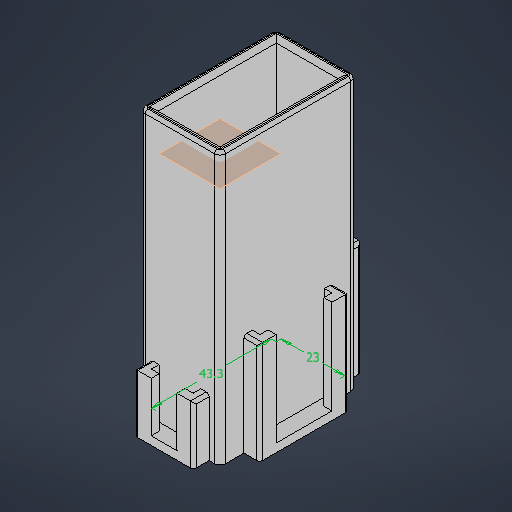
# Autodesk Inventor part: cajaPilas
Saved by Autodesk Inventor 2026.2 (Build 302298010, 298A)
## iProperties
Created: 2026-08-19
Part Number: cajaPilas
Material: Genérico
Document SubType Name: Modeling
Designer: samue
Density: 1 g/cm^3
Appearance: Valor por defecto
Author: samue
Autodesk Inventor part; units mm, degrees
ref_plane "YZ Plane" through (0, 0, 0) normal (1, 0, 0) x (0, 1, 0)
ref_plane "XZ Plane" through (0, 0, 0) normal (0, 1, 0) x (-1, 0, 0)
ref_plane "XY Plane" through (0, 0, 0) normal (0, 0, 1) x (1, 0, 0)
sketch "Boceto1" plane through (0, 0, 0) normal (0, 1, 0) x (-1, 0, 0)
  line L0 (0, 0) -> (23, 0)
  line L1 (23, 0) -> (23, -43.3)
  line L2 (23, -43.3) -> (0, -43.3)
  line L3 (0, -43.3) -> (0, 0)
  dimension "d0" = 23
  dimension "d1" = 43.3
  constraints: 8 end point, 2 parallel, 1 horizontal, 1 perpendicular
  measures "d0" distance of L1.end L2.end
  measures "d1" distance of L0.end L1.end
ref_plane "Plano de trabajo1" through (0, 92, 0) normal (0, 1, 0) x (1, 0, 0)
sketch "Boceto2" plane through (0, 92, 0) normal (0, 1, 0) x (1, 0, 0)
  line L0 (0, 43.3) -> (-23, 43.3) projected
  line L1 (-23, 43.3) -> (-23, 0) projected
  line L2 (-23, 0) -> (0, 0) projected
  line L3 (0, 0) -> (0, 43.3) projected
  line L4 (-26, -1) -> (-26, 44.3)
  line L5 (-24, 46.3) -> (1, 46.3)
  line L6 (3, 44.3) -> (3, -1)
  line L7 (1, -3) -> (-24, -3)
  arc A0 (-26, -1) -> (-24, -3) centre (-24, -1) ccw
  arc A1 (1, -3) -> (3, -1) centre (1, -1) ccw
  arc A2 (3, 44.3) -> (1, 46.3) centre (1, 44.3) ccw
  arc A3 (-24, 46.3) -> (-26, 44.3) centre (-24, 44.3) ccw
  point P0 (-11.5, 21.65)
  point P1 (-26, -3)
  point P2 (-26, 46.3)
  point P3 (3, 46.3)
  point P4 (3, -3)
  dimension "d4" = 21.65
  dimension "d5" = 11.5
  dimension "d6" = 3
  dimension "d9" = 2
  constraints: 8 end point, 8 point on circle, 8 point on line, 8 tangent, 4 centre point, 3 equal radius, 3 other
  measures "d4" distance from line of L0 point (-11.5, 21.65)
  measures "d5" distance from line of L1 point (-11.5, 21.65)
  measures "d6" distance between parallel lines of L1 L4
  measures "d9" radius of A0
extrude "Extrusión2" add sketch "Boceto2" against normal blind 92
sketch "Boceto3" plane through (0, 0, 0) normal (0, -1, 0) x (1, 0, 0)
  line L0 (3, -44.3) -> (3, 1) projected
  arc A0 (3, 1) -> (1, 3) centre (1, 1) ccw projected
  line L1 (1, 3) -> (-24, 3) projected
  arc A1 (-24, 3) -> (-26, 1) centre (-24, 1) ccw projected
  line L2 (-26, 1) -> (-26, -44.3) projected
  arc A2 (-26, -44.3) -> (-24, -46.3) centre (-24, -44.3) ccw projected
  line L3 (-24, -46.3) -> (1, -46.3) projected
  arc A3 (1, -46.3) -> (3, -44.3) centre (1, -44.3) ccw projected
  point P0 (0, 0)
extrude "Extrusión3" add sketch "Boceto3" along normal blind 3
sketch "Boceto4" plane through (0, -3, 0) normal (0, -1, 0) x (1, 0, 0)
  line L0 (3, -44.3) -> (3, 1) projected
  line L1 (3, -8.65) -> (5.8, -8.65)
  line L2 (5.8, -8.65) -> (5.8, -11.55)
  line L3 (5.8, -11.55) -> (8.7, -11.55)
  line L4 (8.7, -11.55) -> (8.7, -5.65)
  line L5 (8.7, -5.65) -> (3, -5.65)
  line L6 (3, -21.65) -> (22.5352, -21.65) construction
  line L7 (3, -34.65) -> (5.8, -34.65)
  line L8 (5.8, -34.65) -> (5.8, -31.75)
  line L9 (5.8, -31.75) -> (8.7, -31.75)
  line L10 (8.7, -31.75) -> (8.7, -37.65)
  line L11 (8.7, -37.65) -> (3, -37.65)
  point P0 (0, 0)
  point P1 (3, -37.65)
  dimension "d12" = 2.8
  dimension "d13" = 2.9
  dimension "d14" = 2.9
  dimension "d15" = 5.9
  dimension "d16" = 13
  constraints: 22 end point, 6 symmetric about line, 4 perpendicular, 2 horizontal, 2 point on line, 1 midpoint
  measures "d12" distance of L1.start L1.end
  measures "d13" distance of L1.end L2.end
  measures "d14" distance of L2.end L3.end
  measures "d15" distance of L3.end L4.end
  measures "d16" distance from line of L6.start L1
extrude "Extrusión4" add sketch "Boceto4" against normal blind 37
sketch "Boceto5" plane through (0, -3, 0) normal (0, -1, 0) x (1, 0, 0)
  line L0 (3, -34.65) -> (3, -8.65) projected
  line L1 (3, -8.65) -> (5.8, -8.65) projected
  line L2 (5.8, -8.65) -> (5.8, -11.55) projected
  line L3 (5.8, -31.75) -> (5.8, -34.65) projected
  line L4 (5.8, -34.65) -> (3, -34.65) projected
  line L5 (5.8, -11.55) -> (8.7, -11.55) projected
  line L6 (8.7, -31.75) -> (5.8, -31.75) projected
  line L7 (8.7, -11.55) -> (8.7, -31.75)
  point P0 (0, 0)
  constraints: 2 end point, 1 vertical
extrude "Extrusión5" add sketch "Boceto5" against normal blind 3
sketch "Boceto6" plane through (0, -3, 0) normal (0, -1, 0) x (1, 0, 0)
  arc A0 (3, 1) -> (1, 3) centre (1, 1) ccw projected
  line L0 (1, 3) -> (-24, 3) projected
  arc A1 (-24, 3) -> (-26, 1) centre (-24, 1) ccw projected
  line L1 (-26, 1) -> (-26, -44.3) projected
  arc A2 (-26, -44.3) -> (-24, -46.3) centre (-24, -44.3) ccw projected
  line L2 (-24, -46.3) -> (1, -46.3) projected
  arc A3 (1, -46.3) -> (3, -44.3) centre (1, -44.3) ccw projected
  line L3 (3, -44.3) -> (3, -37.65) projected
  line L4 (3, -37.65) -> (8.7, -37.65) projected
  line L5 (8.7, -37.65) -> (8.7, -5.65) projected
  line L6 (8.7, -5.65) -> (3, -5.65) projected
  line L7 (3, -5.65) -> (3, 1) projected
  line L8 (0, -43.3) -> (-23, -43.3) projected
  line L9 (3, -8.65) -> (3, -34.65) projected
  point P0 (0, 0)
  point P1 (-11.5, -21.65)
  dimension "d21" = 21.65
  dimension "d22" = 14.5
  measures "d21" distance from line of L8 point (-11.5, -21.65)
  measures "d22" distance from line of L9 point (-11.5, -21.65)
hole "Agujero1" at (-11.5, -3, -21.65) direction (0, 1, 0) diameter 20 end through all
sketch "Boceto7" plane through (0, -3, 0) normal (0, -1, 0) x (1, 0, 0)
  line L0 (1, 3) -> (-24, 3) projected
  line L1 (-3.95, 3) -> (-3.95, 5.8)
  line L2 (-3.95, 5.8) -> (-6.85, 5.8)
  line L3 (-6.85, 5.8) -> (-6.85, 8.7)
  line L4 (-6.85, 8.7) -> (-0.95, 8.7)
  line L5 (-0.95, 8.7) -> (-0.95, 3)
  line L6 (-11.5, 3) -> (-11.5, 18.2857) construction
  line L7 (-19.05, 3) -> (-19.05, 5.8)
  line L8 (-19.05, 5.8) -> (-16.15, 5.8)
  line L9 (-16.15, 5.8) -> (-16.15, 8.7)
  line L10 (-16.15, 8.7) -> (-22.05, 8.7)
  line L11 (-22.05, 8.7) -> (-22.05, 3)
  line L12 (8.7, -11.55) -> (8.7, -31.75) construction
  line L13 (8.7, -21.65) -> (17.1818, -21.65) construction
  line L14 (1, -46.3) -> (-24, -46.3)
  line L15 (-3.95, -46.3) -> (-3.95, -49.1)
  line L16 (-3.95, -49.1) -> (-6.85, -49.1)
  line L17 (-6.85, -49.1) -> (-6.85, -52)
  line L18 (-6.85, -52) -> (-0.95, -52)
  line L19 (-0.95, -52) -> (-0.95, -46.3)
  line L20 (-16.15, -52) -> (-22.05, -52)
  line L21 (-16.15, -49.1) -> (-16.15, -52)
  line L22 (-19.05, -49.1) -> (-16.15, -49.1)
  line L23 (-19.05, -46.3) -> (-19.05, -49.1)
  line L24 (-22.05, -52) -> (-22.05, -46.3)
  point P0 (0, 0)
  dimension "d30" = 2.8
  dimension "d31" = 2.9
  dimension "d32" = 2.9
  dimension "d33" = 5.9
  dimension "d34" = 7.55
  constraints: 46 end point, 20 symmetric about line, 5 perpendicular, 4 point on line, 2 midpoint, 1 horizontal, 1 vertical
  measures "d30" distance of L1.start L1.end
  measures "d31" distance of L1.end L2.end
  measures "d32" distance of L2.end L3.end
  measures "d33" distance of L3.end L4.end
  measures "d34" distance from line of L6.start L1
extrude "Extrusión6" add sketch "Boceto7" against normal blind 21
sketch "Boceto8" plane through (0, -3, 0) normal (0, -1, 0) x (1, 0, 0)
  circle A0 centre (-11.5, -21.65) radius 10 projected
  arc A1 (3, 1) -> (1, 3) centre (1, 1) ccw projected
  line L0 (1, 3) -> (-0.95, 3) projected
  line L1 (-0.95, 3) -> (-0.95, 8.7) projected
  line L2 (-0.95, 8.7) -> (-6.85, 8.7) projected
  line L3 (-6.85, 8.7) -> (-6.85, 5.8) projected
  line L4 (-6.85, 5.8) -> (-3.95, 5.8) projected
  line L5 (-3.95, 5.8) -> (-3.95, 3) projected
  line L6 (-3.95, 3) -> (-19.05, 3) projected
  line L7 (-19.05, 3) -> (-19.05, 5.8) projected
  line L8 (-19.05, 5.8) -> (-16.15, 5.8) projected
  line L9 (-16.15, 5.8) -> (-16.15, 8.7) projected
  line L10 (-16.15, 8.7) -> (-22.05, 8.7) projected
  line L11 (-22.05, 8.7) -> (-22.05, 3) projected
  line L12 (-22.05, 3) -> (-24, 3) projected
  arc A2 (-24, 3) -> (-26, 1) centre (-24, 1) ccw projected
  line L13 (-26, 1) -> (-26, -44.3) projected
  arc A3 (-26, -44.3) -> (-24, -46.3) centre (-24, -44.3) ccw projected
  line L14 (-24, -46.3) -> (-22.05, -46.3) projected
  line L15 (-22.05, -46.3) -> (-22.05, -52) projected
  line L16 (-22.05, -52) -> (-16.15, -52) projected
  line L17 (-16.15, -52) -> (-16.15, -49.1) projected
  line L18 (-16.15, -49.1) -> (-19.05, -49.1) projected
  line L19 (-19.05, -49.1) -> (-19.05, -46.3) projected
  line L20 (-19.05, -46.3) -> (-3.95, -46.3) projected
  line L21 (-3.95, -46.3) -> (-3.95, -49.1) projected
  line L22 (-3.95, -49.1) -> (-6.85, -49.1) projected
  line L23 (-6.85, -49.1) -> (-6.85, -52) projected
  line L24 (-6.85, -52) -> (-0.95, -52) projected
  line L25 (-0.95, -52) -> (-0.95, -46.3) projected
  line L26 (-0.95, -46.3) -> (1, -46.3) projected
  arc A4 (1, -46.3) -> (3, -44.3) centre (1, -44.3) ccw projected
  line L27 (3, -44.3) -> (3, -37.65) projected
  line L28 (3, -37.65) -> (8.7, -37.65) projected
  line L29 (8.7, -37.65) -> (8.7, -5.65) projected
  line L30 (8.7, -5.65) -> (3, -5.65) projected
  line L31 (3, -5.65) -> (3, 1) projected
  line L32 (-6.85, 8.7) -> (-16.15, 8.7)
  line L33 (-6.85, -52) -> (-16.15, -52)
  point P0 (0, 0)
  constraints: 4 end point, 1 horizontal, 1 perpendicular
extrude "Extrusión7" add sketch "Boceto8" against normal blind 3 contours L3 L4 L5 L6 L7 L8 L9 L32
sketch "Boceto9" plane through (0, 92, 0) normal (0, 1, 0) x (1, 0, 0)
  line L0 (3, -1) -> (3, 44.3) projected
  arc A0 (3, 44.3) -> (1, 46.3) centre (1, 44.3) ccw projected
  line L1 (1, 46.3) -> (-24, 46.3) projected
  arc A1 (-24, 46.3) -> (-26, 44.3) centre (-24, 44.3) ccw projected
  line L2 (-26, 44.3) -> (-26, -1) projected
  arc A2 (-26, -1) -> (-24, -3) centre (-24, -1) ccw projected
  line L3 (-24, -3) -> (1, -3) projected
  arc A3 (1, -3) -> (3, -1) centre (1, -1) ccw projected
  line L4 (0, 43.3) -> (0, 0) projected
  line L5 (0, 0) -> (-23, 0) projected
  line L6 (-23, 0) -> (-23, 43.3) projected
  line L7 (-23, 43.3) -> (0, 43.3) projected
extrude "Extrusión8" add sketch "Boceto9" along normal blind 3
fillet "Empalme1" radius 1.5 4 edges at (-11.5, 95, 0) (0, 95, -21.65) (-23, 95, -21.65) (-11.5, 95, -43.3)
fillet "Empalme2" radius 1 8 edges at (2.4142, 95, 2.4142) (3, 95, -21.65) (2.4142, 95, -45.7142) (-11.5, 95, -46.3) (-25.4142, 95, -45.7142) (-26, 95, -21.65) (-25.4142, 95, 2.4142) (-11.5, 95, 3)
sketch "Boceto10" plane through (0, 18, 0) normal (0, 1, 0) x (1, 0, 0)
  line L0 (-0.95, 46.3) -> (-0.95, 52) projected
  line L1 (-0.95, 52) -> (-6.85, 52) projected
  line L2 (-6.85, 52) -> (-6.85, 49.1) projected
  line L3 (-6.85, 49.1) -> (-3.95, 49.1) projected
  line L4 (-3.95, 49.1) -> (-3.95, 46.3) projected
  line L5 (-0.95, 46.3) -> (-3.95, 46.3) projected
  line L6 (-16.15, 49.1) -> (-16.15, 52) projected
  line L7 (-16.15, 52) -> (-22.05, 52) projected
  line L8 (-22.05, 52) -> (-22.05, 46.3) projected
  line L9 (-19.05, 46.3) -> (-22.05, 46.3) projected
  line L10 (-19.05, 46.3) -> (-19.05, 49.1) projected
  line L11 (-19.05, 49.1) -> (-16.15, 49.1) projected
  point P0 (0, 0)
extrude "Extrusión9" add sketch "Boceto10" along normal blind 20
fillet "Empalme3" radius 1 12 edges at (8.7, 15.5, -37.65) (8.7, 15.5, -5.65) (-0.95, 7.5, 8.7) (-22.05, 7.5, 8.7) (5.85, 34, -37.65) (5.85, 34, -5.65) (-0.95, 18, 5.85) (-22.05, 18, 5.85) (-0.95, 17.5, -52) (-0.95, 38, -49.15) (-22.05, 17.5, -52) (-22.05, 38, -49.15)
